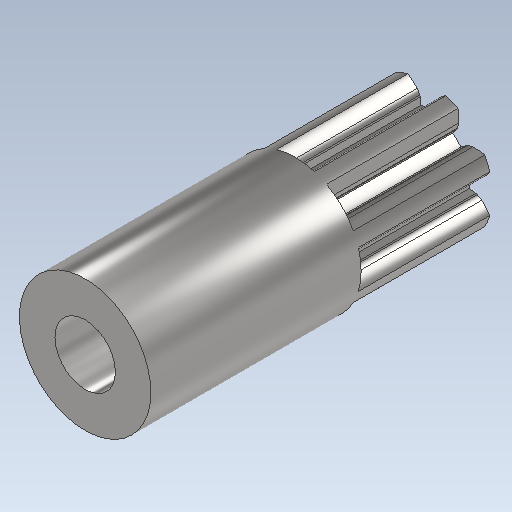
# Autodesk Inventor part: マブチRS-380PHピニオン
Saved by Autodesk Inventor 2020.2 (Build 242310000, 310)
## iProperties
Created: 2020-02-11
Part Number: マブチRS-380PHピニオン
Material: 鋼、炭素鋼
Document SubType Name: Modeling
Designer: aoyam
Density: 7.85 g/cm^3
Appearance: 半つや出し
Mass: 1.36693 g
Surface Area: 3.66361 cm^2
Volume: 0.174131 cm^3
Author: aoyam
Autodesk Inventor part; units mm, degrees
ref_plane "YZ Plane" through (0, 0, 0) normal (1, 0, 0) x (0, 1, 0)
ref_plane "XZ Plane" through (0, 0, 0) normal (0, 1, 0) x (-1, 0, 0)
ref_plane "XY Plane" through (0, 0, 0) normal (0, 0, 1) x (1, 0, 0)
sketch "スケッチ1" plane through (0, 0, 0) normal (0, 0, 1) x (1, 0, 0)
  arc A0 (1.3221, 2.5189) -> (1.3056, 2.4652) centre (1.5585, 2.4166) ccw
  arc A1 (1.423, 2.6891) -> (1.3221, 2.5189) centre (1.989, 2.2385) ccw
  arc A2 (1.7731, 2.9966) -> (1.423, 2.6891) centre (2.4499, 1.873) ccw
  arc A3 (-0.112, 2.1496) -> (-0.0857, 2.0999) centre (0.1275, 2.2444) ccw
  arc A4 (-0.161, 2.3413) -> (-0.112, 2.1496) centre (0.5579, 2.4229) ccw
  arc A5 (-0.1308, 2.8063) -> (-0.161, 2.3413) centre (1.1423, 2.4904) ccw
  arc A6 (-0.8649, 0.8744) -> (-0.8112, 0.8579) centre (-0.7626, 1.1108) ccw
  arc A7 (-1.0351, 0.9754) -> (-0.8649, 0.8744) centre (-0.5845, 1.5413) ccw
  arc A8 (-1.3426, 1.3254) -> (-1.0351, 0.9754) centre (-0.219, 2.0023) ccw
  arc A9 (-0.4956, -0.5597) -> (-0.4459, -0.5334) centre (-0.5904, -0.3202) ccw
  arc A10 (-0.6873, -0.6086) -> (-0.4956, -0.5597) centre (-0.7689, 0.1102) ccw
  arc A11 (-1.1523, -0.5785) -> (-0.6873, -0.6086) centre (-0.8364, 0.6946) ccw
  arc A12 (0.7796, -1.3126) -> (0.7961, -1.2589) centre (0.5432, -1.2103) ccw
  arc A13 (0.6786, -1.4828) -> (0.7796, -1.3126) centre (0.1127, -1.0321) ccw
  arc A14 (0.3286, -1.7902) -> (0.6786, -1.4828) centre (-0.3483, -0.6666) ccw
  arc A15 (2.2137, -0.9433) -> (2.1874, -0.8936) centre (1.9742, -1.0381) ccw
  arc A16 (2.2626, -1.135) -> (2.2137, -0.9433) centre (1.5438, -1.2166) ccw
  arc A17 (2.2325, -1.5999) -> (2.2626, -1.135) centre (0.9594, -1.284) ccw
  arc A18 (2.9666, 0.3319) -> (2.9129, 0.3484) centre (2.8643, 0.0955) ccw
  arc A19 (3.1368, 0.231) -> (2.9666, 0.3319) centre (2.6861, -0.335) ccw
  arc A20 (3.4442, -0.1191) -> (3.1368, 0.231) centre (2.3206, -0.7959) ccw
  arc A21 (2.5973, 1.766) -> (2.5476, 1.7397) centre (2.6921, 1.5265) ccw
  arc A22 (2.789, 1.815) -> (2.5973, 1.766) centre (2.8706, 1.0961) ccw
  arc A23 (3.2539, 1.7848) -> (2.789, 1.815) centre (2.938, 0.5117) ccw
  arc A24 (0.7961, 2.4652) -> (0.7796, 2.5189) centre (0.5432, 2.4166) ccw
  arc A25 (0.7796, 2.5189) -> (0.6786, 2.6891) centre (0.1127, 2.2385) ccw
  arc A26 (0.6786, 2.6891) -> (0.3286, 2.9966) centre (-0.3483, 1.873) ccw
  arc A27 (-0.4459, 1.7397) -> (-0.4956, 1.766) centre (-0.5904, 1.5265) ccw
  arc A28 (-0.4956, 1.766) -> (-0.6873, 1.815) centre (-0.7689, 1.0961) ccw
  arc A29 (-0.6873, 1.815) -> (-1.1523, 1.7848) centre (-0.8364, 0.5117) ccw
  arc A30 (-0.8112, 0.3484) -> (-0.8649, 0.3319) centre (-0.7626, 0.0955) ccw
  arc A31 (-0.8649, 0.3319) -> (-1.0351, 0.231) centre (-0.5845, -0.335) ccw
  arc A32 (-1.0351, 0.231) -> (-1.3426, -0.1191) centre (-0.219, -0.7959) ccw
  arc A33 (-0.0857, -0.8936) -> (-0.112, -0.9433) centre (0.1275, -1.0381) ccw
  arc A34 (-0.112, -0.9433) -> (-0.161, -1.135) centre (0.5579, -1.2166) ccw
  arc A35 (-0.161, -1.135) -> (-0.1308, -1.5999) centre (1.1423, -1.284) ccw
  arc A36 (1.3056, -1.2589) -> (1.3221, -1.3126) centre (1.5585, -1.2103) ccw
  arc A37 (1.3221, -1.3126) -> (1.423, -1.4828) centre (1.989, -1.0321) ccw
  arc A38 (1.423, -1.4828) -> (1.7731, -1.7902) centre (2.4499, -0.6666) ccw
  arc A39 (2.5476, -0.5334) -> (2.5973, -0.5597) centre (2.6921, -0.3202) ccw
  arc A40 (2.5973, -0.5597) -> (2.789, -0.6086) centre (2.8706, 0.1102) ccw
  arc A41 (2.789, -0.6086) -> (3.2539, -0.5785) centre (2.938, 0.6946) ccw
  arc A42 (2.9129, 0.8579) -> (2.9666, 0.8744) centre (2.8643, 1.1108) ccw
  arc A43 (2.9666, 0.8744) -> (3.1368, 0.9754) centre (2.6861, 1.5413) ccw
  arc A44 (3.1368, 0.9754) -> (3.4442, 1.3254) centre (2.3206, 2.0023) ccw
  arc A45 (2.1874, 2.0999) -> (2.2137, 2.1496) centre (1.9742, 2.2444) ccw
  arc A46 (2.2137, 2.1496) -> (2.2626, 2.3413) centre (1.5438, 2.4229) ccw
  arc A47 (2.2626, 2.3413) -> (2.2325, 2.8063) centre (0.9594, 2.4904) ccw
  arc A48 (1.2711, 2.2132) -> (0.8306, 2.2132) centre (1.0508, 0.6032) ccw
  arc A49 (0.0681, 1.8973) -> (-0.2433, 1.5859) centre (1.0508, 0.6032) ccw
  arc A50 (-0.5592, 0.8234) -> (-0.5592, 0.3829) centre (1.0508, 0.6032) ccw
  arc A51 (-0.2433, -0.3796) -> (0.0681, -0.691) centre (1.0508, 0.6032) ccw
  arc A52 (0.8306, -1.0068) -> (1.2711, -1.0068) centre (1.0508, 0.6032) ccw
  arc A53 (2.0336, -0.691) -> (2.345, -0.3796) centre (1.0508, 0.6032) ccw
  arc A54 (2.6608, 0.3829) -> (2.6608, 0.8234) centre (1.0508, 0.6032) ccw
  arc A55 (2.345, 1.5859) -> (2.0336, 1.8973) centre (1.0508, 0.6032) ccw
  arc A56 (0.3286, 2.9966) -> (-0.1308, 2.8063) centre (1.0508, 0.6032) ccw
  arc A57 (-1.1523, 1.7848) -> (-1.3426, 1.3254) centre (1.0508, 0.6032) ccw
  arc A58 (-1.3426, -0.1191) -> (-1.1523, -0.5785) centre (1.0508, 0.6032) ccw
  arc A59 (-0.1308, -1.5999) -> (0.3286, -1.7902) centre (1.0508, 0.6032) ccw
  arc A60 (1.7731, -1.7902) -> (2.2325, -1.5999) centre (1.0508, 0.6032) ccw
  arc A61 (3.2539, -0.5785) -> (3.4442, -0.1191) centre (1.0508, 0.6032) ccw
  arc A62 (3.4442, 1.3254) -> (3.2539, 1.7848) centre (1.0508, 0.6032) ccw
  arc A63 (2.2325, 2.8063) -> (1.7731, 2.9966) centre (1.0508, 0.6032) ccw
  line L0 (1.2711, 2.2132) -> (1.3056, 2.4652)
  line L1 (0.0681, 1.8973) -> (-0.0857, 2.0999)
  line L2 (-0.5592, 0.8234) -> (-0.8112, 0.8579)
  line L3 (-0.2433, -0.3796) -> (-0.4459, -0.5334)
  line L4 (0.8306, -1.0068) -> (0.7961, -1.2589)
  line L5 (2.0336, -0.691) -> (2.1874, -0.8936)
  line L6 (2.6608, 0.3829) -> (2.9129, 0.3484)
  line L7 (2.345, 1.5859) -> (2.5476, 1.7397)
  line L8 (0.8306, 2.2132) -> (0.7961, 2.4652)
  line L9 (-0.2433, 1.5859) -> (-0.4459, 1.7397)
  line L10 (-0.5592, 0.3829) -> (-0.8112, 0.3484)
  line L11 (0.0681, -0.691) -> (-0.0857, -0.8936)
  line L12 (1.2711, -1.0068) -> (1.3056, -1.2589)
  line L13 (2.345, -0.3796) -> (2.5476, -0.5334)
  line L14 (2.6608, 0.8234) -> (2.9129, 0.8579)
  line L15 (2.0336, 1.8973) -> (2.1874, 2.0999)
  line L16 (-3.4492, 0.6032) -> (5.5508, 0.6032)
  line L17 (1.0508, -3.8968) -> (1.0508, 5.1032)
  circle A64 centre (1.0508, 0.6032) radius 1.15
  point P0 (0, 0)
  point P1 (-0.8112, 0.8579)
  point P2 (-0.5592, 0.8234)
  point P3 (-0.5592, 0.3829)
  point P4 (-0.8611, 0.3335)
  point P5 (-1.034, 0.2319)
  point P6 (-1.3426, -0.1191)
  point P7 (-1.1523, -0.5785)
  point P8 (-0.6859, -0.6085)
  point P9 (-0.4918, -0.5581)
  point P10 (-0.1104, -0.9395)
  point P11 (-0.1608, -1.1336)
  point P12 (-0.1308, -1.5999)
  point P13 (0.3286, -1.7902)
  point P14 (0.6795, -1.4816)
  point P15 (0.7812, -1.3088)
  point P16 (0.7961, -1.2589)
  point P17 (0.8306, -1.0068)
  point P18 (1.2711, -1.0068)
  point P19 (1.3205, -1.3088)
  point P20 (1.4221, -1.4816)
  point P21 (1.7731, -1.7902)
  point P22 (2.2325, -1.5999)
  point P23 (2.2625, -1.1336)
  point P24 (2.2121, -0.9395)
  point P25 (2.5935, -0.5581)
  point P26 (2.7876, -0.6085)
  point P27 (3.2539, -0.5785)
  point P28 (3.1356, 0.2319)
  point P29 (2.9628, 0.3335)
  point P30 (2.9129, 0.3484)
  point P31 (2.6608, 0.3829)
  point P32 (2.6608, 0.8234)
  point P33 (2.9628, 0.8728)
  point P34 (3.1356, 0.9745)
  point P35 (3.4442, 1.3254)
  point P36 (3.2539, 1.7848)
  point P37 (2.7876, 1.8148)
  point P38 (2.5935, 1.7644)
  point P39 (2.2121, 2.1458)
  point P40 (2.2625, 2.3399)
  point P41 (2.2325, 2.8063)
  point P42 (1.7731, 2.9966)
  point P43 (1.4221, 2.688)
  point P44 (1.3205, 2.5151)
  point P45 (1.3056, 2.4652)
  point P46 (0.8306, 2.2132)
  point P47 (0.7812, 2.5151)
  point P48 (0.6795, 2.688)
  point P49 (0.3286, 2.9966)
  point P50 (-0.1308, 2.8063)
  point P51 (-0.1608, 2.3399)
  point P52 (-0.1104, 2.1458)
  point P53 (-0.4918, 1.7644)
  point P54 (-0.6859, 1.8148)
  point P55 (-1.1523, 1.7848)
  point P56 (-1.3426, 1.3254)
  point P57 (-1.034, 0.9745)
  point P58 (-0.8611, 0.8728)
  point P59 (1.3205, -1.3088)
  point P60 (1.4221, -1.4816)
  point P61 (2.2625, -1.1336)
  point P62 (2.2137, -0.9433)
  point P63 (2.5935, -0.5581)
  point P64 (2.7876, -0.6085)
  point P65 (3.1356, 0.2319)
  point P66 (2.9628, 0.8728)
  point P67 (3.1356, 0.9745)
  point P68 (2.789, 1.815)
  point P69 (2.5935, 1.7644)
  point P70 (2.2137, 2.1496)
  point P71 (2.2626, 2.3413)
  point P72 (1.423, 2.6891)
  point P73 (1.3221, 2.5189)
  point P74 (0.7796, 2.5189)
  point P75 (0.6795, 2.688)
  point P76 (-0.1608, 2.3399)
  point P77 (-0.1104, 2.1458)
  point P78 (-0.4956, 1.766)
  point P79 (-0.6859, 1.8148)
  point P80 (-1.0351, 0.9754)
  point P81 (-0.8611, 0.8728)
  point P82 (-0.8649, 0.3319)
  point P83 (-1.0351, 0.231)
  point P84 (-0.6873, -0.6086)
  point P85 (-0.4918, -0.5581)
  point P86 (-0.1104, -0.9395)
  point P87 (-0.1608, -1.1336)
  point P88 (0.6786, -1.4828)
  point P89 (0.7812, -1.3088)
  dimension "d2" = 2.3
  constraints: 128 point on circle, 65 centre point, 36 end point, 1 coincident
  measures "d2" diameter of A64
extrude "押し出し1" add sketch "スケッチ1" along normal blind 5 contours A1 A2 A63 A47 A46 A45 L15 A55 L7 A21 A22 A23 A62 A44 A43 A42 L14 A54 L16 A64 L17 A48 L0 A0 | L17 A64 L16 A50 L2 A6 A7 A8 A57 A29 A28 A27 L9 A49 L1 A3 A4 A5 A56 A26 A25 A24 L8 A48 | L16 A54 L6 A18 A19 A20 A61 A41 A40 A39 L13 A53 L5 A15 A16 A17 A60 A38 A37 A36 L12 A52 L17 A64 | A64 L17 A52 L4 A12 A13 A14 A59 A35 A34 A33 L11 A51 L3 A9 A10 A11 A58 A32 A31 A30 L10 A50 L16
sketch "スケッチ2" plane through (0, 0, 5) normal (0, 0, 1) x (1, 0, 0)
  arc A0 (3.2539, 1.7848) -> (2.789, 1.815) centre (2.938, 0.5117) ccw projected
  arc A1 (2.789, 1.815) -> (2.5973, 1.766) centre (2.8706, 1.0961) ccw projected
  arc A2 (2.5973, 1.766) -> (2.5476, 1.7397) centre (2.6921, 1.5265) ccw projected
  line L0 (2.5476, 1.7397) -> (2.345, 1.5859) projected
  arc A3 (2.345, 1.5859) -> (2.0336, 1.8973) centre (1.0508, 0.6032) ccw projected
  line L1 (2.0336, 1.8973) -> (2.1874, 2.0999) projected
  arc A4 (2.1874, 2.0999) -> (2.2137, 2.1496) centre (1.9742, 2.2444) ccw projected
  arc A5 (2.2137, 2.1496) -> (2.2626, 2.3413) centre (1.5438, 2.4229) ccw projected
  arc A6 (2.2626, 2.3413) -> (2.2325, 2.8063) centre (0.9594, 2.4904) ccw projected
  arc A7 (2.2325, 2.8063) -> (1.7731, 2.9966) centre (1.0508, 0.6032) ccw projected
  arc A8 (1.7731, 2.9966) -> (1.423, 2.6891) centre (2.4499, 1.873) ccw projected
  arc A9 (1.423, 2.6891) -> (1.3221, 2.5189) centre (1.989, 2.2385) ccw projected
  arc A10 (1.3221, 2.5189) -> (1.3056, 2.4652) centre (1.5585, 2.4166) ccw projected
  line L2 (1.3056, 2.4652) -> (1.2711, 2.2132) projected
  arc A11 (1.2711, 2.2132) -> (0.8306, 2.2132) centre (1.0508, 0.6032) ccw projected
  line L3 (0.8306, 2.2132) -> (0.7961, 2.4652) projected
  arc A12 (0.7961, 2.4652) -> (0.7796, 2.5189) centre (0.5432, 2.4166) ccw projected
  arc A13 (0.7796, 2.5189) -> (0.6795, 2.688) centre (0.1127, 2.2385) ccw projected
  arc A14 (0.6795, 2.688) -> (0.3286, 2.9966) centre (-0.3483, 1.873) ccw projected
  arc A15 (0.3286, 2.9966) -> (-0.1308, 2.8063) centre (1.0508, 0.6032) ccw projected
  arc A16 (-0.1308, 2.8063) -> (-0.161, 2.3413) centre (1.1423, 2.4904) ccw projected
  arc A17 (-0.161, 2.3413) -> (-0.112, 2.1496) centre (0.5579, 2.4229) ccw projected
  arc A18 (-0.112, 2.1496) -> (-0.0857, 2.0999) centre (0.1275, 2.2444) ccw projected
  line L4 (-0.0857, 2.0999) -> (0.0681, 1.8973) projected
  arc A19 (0.0681, 1.8973) -> (-0.2433, 1.5859) centre (1.0508, 0.6032) ccw projected
  line L5 (-0.2433, 1.5859) -> (-0.4459, 1.7397) projected
  arc A20 (-0.4459, 1.7397) -> (-0.4956, 1.766) centre (-0.5904, 1.5265) ccw projected
  arc A21 (-0.4956, 1.766) -> (-0.6859, 1.8148) centre (-0.7689, 1.0961) ccw projected
  arc A22 (-0.6859, 1.8148) -> (-1.1523, 1.7848) centre (-0.8364, 0.5117) ccw projected
  arc A23 (-1.1523, 1.7848) -> (-1.3426, 1.3254) centre (1.0508, 0.6032) ccw projected
  arc A24 (-1.3426, 1.3254) -> (-1.0351, 0.9754) centre (-0.219, 2.0023) ccw projected
  arc A25 (-1.0351, 0.9754) -> (-0.8649, 0.8744) centre (-0.5845, 1.5413) ccw projected
  arc A26 (-0.8649, 0.8744) -> (-0.8112, 0.8579) centre (-0.7626, 1.1108) ccw projected
  line L6 (-0.8112, 0.8579) -> (-0.5592, 0.8234) projected
  arc A27 (-0.5592, 0.8234) -> (-0.5592, 0.3829) centre (1.0508, 0.6032) ccw projected
  line L7 (-0.5592, 0.3829) -> (-0.8112, 0.3484) projected
  arc A28 (-0.8112, 0.3484) -> (-0.8649, 0.3319) centre (-0.7626, 0.0955) ccw projected
  arc A29 (-0.8649, 0.3319) -> (-1.0351, 0.231) centre (-0.5845, -0.335) ccw projected
  arc A30 (-1.0351, 0.231) -> (-1.3426, -0.1191) centre (-0.219, -0.7959) ccw projected
  arc A31 (-1.3426, -0.1191) -> (-1.1523, -0.5785) centre (1.0508, 0.6032) ccw projected
  arc A32 (-1.1523, -0.5785) -> (-0.6873, -0.6086) centre (-0.8364, 0.6946) ccw projected
  arc A33 (-0.6873, -0.6086) -> (-0.4956, -0.5597) centre (-0.7689, 0.1102) ccw projected
  arc A34 (-0.4956, -0.5597) -> (-0.4459, -0.5334) centre (-0.5904, -0.3202) ccw projected
  line L8 (-0.4459, -0.5334) -> (-0.2433, -0.3796) projected
  arc A35 (-0.2433, -0.3796) -> (0.0681, -0.691) centre (1.0508, 0.6032) ccw projected
  line L9 (0.0681, -0.691) -> (-0.0857, -0.8936) projected
  arc A36 (-0.0857, -0.8936) -> (-0.1104, -0.9395) centre (0.1275, -1.0381) ccw projected
  arc A37 (-0.1104, -0.9395) -> (-0.1608, -1.1336) centre (0.5579, -1.2166) ccw projected
  arc A38 (-0.1608, -1.1336) -> (-0.1308, -1.5999) centre (1.1423, -1.284) ccw projected
  arc A39 (-0.1308, -1.5999) -> (0.3286, -1.7902) centre (1.0508, 0.6032) ccw projected
  arc A40 (0.3286, -1.7902) -> (0.6786, -1.4828) centre (-0.3483, -0.6666) ccw projected
  arc A41 (0.6786, -1.4828) -> (0.7796, -1.3126) centre (0.1127, -1.0321) ccw projected
  arc A42 (0.7796, -1.3126) -> (0.7961, -1.2589) centre (0.5432, -1.2103) ccw projected
  line L10 (0.7961, -1.2589) -> (0.8306, -1.0068) projected
  arc A43 (0.8306, -1.0068) -> (1.2711, -1.0068) centre (1.0508, 0.6032) ccw projected
  line L11 (1.2711, -1.0068) -> (1.3056, -1.2589) projected
  arc A44 (1.3056, -1.2589) -> (1.3205, -1.3088) centre (1.5585, -1.2103) ccw projected
  arc A45 (1.3205, -1.3088) -> (1.4221, -1.4816) centre (1.989, -1.0321) ccw projected
  arc A46 (1.4221, -1.4816) -> (1.7731, -1.7902) centre (2.4499, -0.6666) ccw projected
  arc A47 (1.7731, -1.7902) -> (2.2325, -1.5999) centre (1.0508, 0.6032) ccw projected
  arc A48 (2.2325, -1.5999) -> (2.2626, -1.135) centre (0.9594, -1.284) ccw projected
  arc A49 (2.2626, -1.135) -> (2.2137, -0.9433) centre (1.5438, -1.2166) ccw projected
  arc A50 (2.2137, -0.9433) -> (2.1874, -0.8936) centre (1.9742, -1.0381) ccw projected
  line L12 (2.1874, -0.8936) -> (2.0336, -0.691) projected
  arc A51 (2.0336, -0.691) -> (2.345, -0.3796) centre (1.0508, 0.6032) ccw projected
  line L13 (2.345, -0.3796) -> (2.5476, -0.5334) projected
  arc A52 (2.5476, -0.5334) -> (2.5935, -0.5581) centre (2.6921, -0.3202) ccw projected
  arc A53 (2.5935, -0.5581) -> (2.7876, -0.6085) centre (2.8706, 0.1102) ccw projected
  arc A54 (2.7876, -0.6085) -> (3.2539, -0.5785) centre (2.938, 0.6946) ccw projected
  arc A55 (3.2539, -0.5785) -> (3.4442, -0.1191) centre (1.0508, 0.6032) ccw projected
  arc A56 (3.4442, -0.1191) -> (3.1368, 0.231) centre (2.3206, -0.7959) ccw projected
  arc A57 (3.1368, 0.231) -> (2.9666, 0.3319) centre (2.6861, -0.335) ccw projected
  arc A58 (2.9666, 0.3319) -> (2.9129, 0.3484) centre (2.8643, 0.0955) ccw projected
  line L14 (2.9129, 0.3484) -> (2.6608, 0.3829) projected
  arc A59 (2.6608, 0.3829) -> (2.6608, 0.8234) centre (1.0508, 0.6032) ccw projected
  line L15 (2.6608, 0.8234) -> (2.9129, 0.8579) projected
  arc A60 (2.9129, 0.8579) -> (2.9628, 0.8728) centre (2.8643, 1.1108) ccw projected
  arc A61 (2.9628, 0.8728) -> (3.1356, 0.9745) centre (2.6861, 1.5413) ccw projected
  arc A62 (3.1356, 0.9745) -> (3.4442, 1.3254) centre (2.3206, 2.0023) ccw projected
  arc A63 (3.4442, 1.3254) -> (3.2539, 1.7848) centre (1.0508, 0.6032) ccw projected
  circle A64 centre (1.0508, 0.6032) radius 1.15 projected
  circle A65 centre (1.0508, 0.6032) radius 2.5
  point P0 (0, 0)
  point P1 (3.4442, 1.3254)
  point P2 (3.2539, 1.7848)
  point P3 (2.2325, 2.8063)
  point P4 (1.7731, 2.9966)
  point P5 (0.3286, 2.9966)
  point P6 (-0.1308, 2.8063)
  point P7 (-1.1523, 1.7848)
  point P8 (-1.3426, 1.3254)
  point P9 (-1.3426, -0.1191)
  point P10 (-1.1523, -0.5785)
  point P11 (-0.1308, -1.5999)
  point P12 (0.3286, -1.7902)
  point P13 (1.7731, -1.7902)
  point P14 (2.2325, -1.5999)
  point P15 (3.2539, -0.5785)
  point P16 (3.4442, -0.1191)
  constraints: 1 centre point, 1 concentric, 8 other
extrude "押し出し2" add sketch "スケッチ2" along normal blind 8 contours A63 A62 A61 A60 L15 A59 L14 A58 A57 A56 A55 A54 A53 A52 L13 A51 L12 A50 A49 A48 A47 A46 A45 A44 L11 A43 L10 A42 A41 A40 A39 A38 A37 A36 L9 A35 L8 A34 A33 A32 A31 A30 A29 A28 L7 A27 L6 A26 A25 A24 A23 A22 A21 A20 L5 A19 L4 A18 A17 A16 A15 A14 A13 A12 L3 A11 L2 A10 A9 A8 A7 A6 A5 A4 L1 A3 L0 A2 A1 A0 | A0 A1 A2 L0 A3 L1 A4 A5 A6 A65 | A65 A56 A57 A58 L14 A59 L15 A60 A61 A62 | A8 A9 A10 L2 A11 L3 A12 A13 A14 A65 | A65 A48 A49 A50 L12 A51 L13 A52 A53 A54 | A16 A17 A18 L4 A19 L5 A20 A21 A22 A65 | A65 A40 A41 A42 L10 A43 L11 A44 A45 A46 | A24 A25 A26 L6 A27 L7 A28 A29 A30 A65 | A65 A32 A33 A34 L8 A35 L9 A36 A37 A38 | A64
sketch "スケッチ3" plane through (1.0508, 0.6032, 13) normal (0, 0, 1) x (1, 0, 0)
  circle A0 centre (0, 0) radius 1.15
  point P0 (-1.0508, -0.6032)
  dimension "d5" = 2.3
  constraints: 1 centre point
  measures "d5" diameter of A0
extrude "押し出し3" cut sketch "スケッチ3" against normal blind 13
